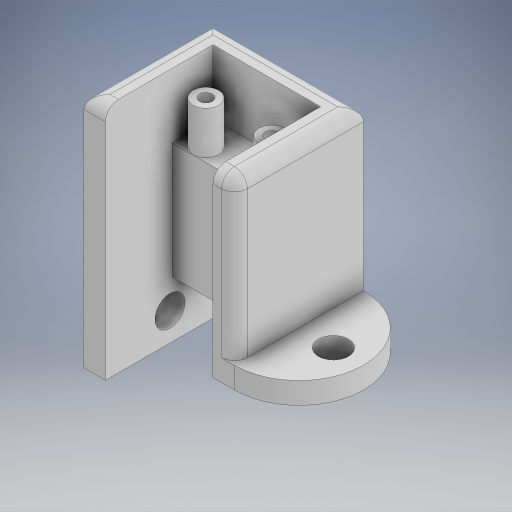
# Autodesk Inventor part: imu_mount
Saved by Autodesk Inventor 2024 (Build 280153000, 153)
## iProperties
Created: 2025-01-15
Part Number: imu_mount
Material: Generic
Document SubType Name: Modeling
Designer: Alex
Density: 1 g/cm^3
Appearance: Default
Author: Alex
Autodesk Inventor part; units mm, degrees
ref_plane "YZ Plane" through (0, 0, 0) normal (1, 0, 0) x (0, 1, 0)
ref_plane "XZ Plane" through (0, 0, 0) normal (0, 1, 0) x (-1, 0, 0)
ref_plane "XY Plane" through (0, 0, 0) normal (0, 0, 1) x (1, 0, 0)
sketch "Sketch1" plane through (0, 0, 0) normal (0, 1, 0) x (-1, 0, 0)
  line L0 (0, 0) -> (35, 0) construction
  line L1 (35, 0) -> (35, -30)
  line L2 (35, -30) -> (0, -30)
  line L3 (0, -30) -> (0, 0)
  line L4 (30, -25) -> (30, -5)
  line L5 (30, -5) -> (5, -5) construction
  line L6 (5, -5) -> (5, -25)
  line L7 (5, -25) -> (30, -25)
  line L8 (30, -5) -> (30, 0)
  line L9 (5, -5) -> (5, 0)
  line L10 (5, 0) -> (0, 0)
  line L11 (30, 0) -> (35, 0)
  dimension "d0" = 35
  dimension "d1" = 30
  dimension "d2" = 5
  constraints: 24 end point, 4 parallel, 4 perpendicular, 2 collinear, 2 point on line, 1 horizontal, 3 other
  measures "d0" distance between parallel lines of L3 L1
  measures "d1" distance between parallel lines of L2 L0
  measures "d2" distance between parallel lines of L1 L4
extrude "Extrusion1" add sketch "Sketch1" along normal blind 42
sketch "Sketch2" plane through (0, 0, 0) normal (0, 1, 0) x (-1, 0, 0)
  line L0 (30, 0) -> (30, -25) projected
  line L1 (5, -25) -> (5, 0) projected
  line L2 (30, -25) -> (5, -25)
  line L3 (5, -25) -> (5, -15.519)
  line L4 (5, -15.519) -> (30, -15.519)
  line L5 (30, -15.519) -> (30, -25)
  point P0 (0, 0)
  dimension "d5" = 9.481
  constraints: 8 end point, 2 parallel, 1 horizontal, 1 perpendicular, 1 point on line
  measures "d5" distance between parallel lines of L2 L4
extrude "Extrusion2" add sketch "Sketch2" along normal blind 27
sketch "Sketch3" plane through (0, 27, 0) normal (0, 1, 0) x (1, 0, 0)
  circle A0 centre (-25.15, 18.519) radius 1.5
  line L0 (-30, 0) -> (-30, 15.519) projected
  circle A1 centre (-25.15, 18.519) radius 3
  line L1 (-30, 15.519) -> (-5, 15.519) projected
  line L2 (-17.5, 15.519) -> (-17.5, 30) construction
  line L3 (0, 30) -> (-35, 30) construction
  circle A2 centre (-9.85, 18.519) radius 1.5
  circle A3 centre (-9.85, 18.519) radius 3
  point P0 (0, 0)
  dimension "d8" = 3
  dimension "d9" = 4.85
  dimension "d10" = 6
  constraints: 4 centre point, 2 coincident, 2 end point, 2 midpoint, 2 symmetric about line, 1 tangent, 2 other
  measures "d8" diameter of A0
  measures "d9" distance from line of L0 A0.centre
  measures "d10" diameter of A1
extrude "Extrusion3" add sketch "Sketch3" along normal blind 10
sketch "Sketch4" plane through (0, 0, 0) normal (0, -1, 0) x (1, 0, 0)
  line L0 (-35, -30) -> (-35, 0) projected
  line L1 (0, -30) -> (-35, -30) projected
  line L2 (-35, 0) -> (-30, 0)
  line L3 (-30, 0) -> (-30, -30)
  line L4 (-30, -30) -> (-35, -30)
  line L5 (-35, -30) -> (-35, 0)
  line L6 (-30, 0) -> (-30, -15.519) projected
  point P0 (0, 0)
  constraints: 8 end point, 2 parallel, 2 point on line, 1 horizontal, 1 perpendicular
extrude "Extrusion4" add sketch "Sketch4" along normal blind 13.047
sketch "Sketch5" plane through (0, 0, 0) normal (1, 0, 0) x (0, 0, -1)
  line L0 (15.519, 0) -> (0, 0) projected
  line L1 (30, 0) -> (30, 42) projected
  line L2 (0, 0) -> (30, 0)
  line L3 (30, 0) -> (30, 5)
  line L4 (30, 5) -> (0, 5)
  line L5 (0, 5) -> (0, 0)
  dimension "d15" = 5
  constraints: 8 end point, 2 parallel, 1 horizontal, 1 perpendicular, 1 point on line
  measures "d15" distance between parallel lines of L2 L4
extrude "Extrusion5" add sketch "Sketch5" along normal blind 15
sketch "Sketch6" plane through (0, 5, 0) normal (0, 1, 0) x (1, 0, 0)
  circle A0 centre (8, 7) radius 3.5 construction
  circle A1 centre (8, 23) radius 3.5 construction
  line L0 (8, 7) -> (8, 23) construction
  line L1 (8, 15) -> (15, 15) construction
  line L2 (15, 0) -> (15, 30) construction
  line L3 (15, 30) -> (15, 0) construction
  line L4 (0, 30) -> (15, 30) construction
  circle A2 centre (8, 15) radius 3.5
  point P0 (0, 0)
  dimension "d18" = 7
  dimension "d19" = 7
  dimension "d20" = 7
  dimension "d21" = 7
  dimension "d25" = 7
  constraints: 4 end point, 3 centre point, 2 midpoint, 2 perpendicular, 1 coincident
  measures "d18" diameter of A0
  measures "d19" diameter of A1
  measures "d20" distance from line of L2 L0.end
  measures "d21" distance from line of L4 L0.end
  measures "d25" diameter of A2
extrude "Extrusion6" cut sketch "Sketch6" against normal up to surface (5 mm away) from surface at 0
sketch "Sketch7" plane through (-35, 42, -30) normal (-1, 0, 0) x (0, 0, 1)
  point P0 (30, -42)
sketch "Sketch8" plane through (-35, 42, -30) normal (-1, 0, 0) x (0, 0, 1)
  line L0 (0, -55.047) -> (0, 0) projected
  line L1 (30, -55.047) -> (30, 0) projected
  line L2 (0, -55.047) -> (30, -55.047) construction
  line L3 (30, -55.047) -> (30, -42.047) construction
  line L4 (30, -42.047) -> (0, -42.047) construction
  line L5 (0, -42.047) -> (0, -55.047) construction
  circle A0 centre (15, -48.547) radius 3.5
  point P0 (30, -42)
  dimension "d24" = 13
  dimension "d26" = 7
  dimension "d27" = 6.5
  dimension "d28" = 15
  constraints: 8 end point, 2 parallel, 1 centre point, 1 horizontal, 1 perpendicular, 1 point on line
  measures "d24" distance of L3.end L2.end
  measures "d26" diameter of A0
  measures "d27" distance from line of L2 A0.centre
  measures "d28" distance from line of L0 A0.centre
extrude "Extrusion7" cut sketch "Sketch8" against normal up to next
fillet "Fillet1" radius 3 6 edges at (0, 42, -15) (0, 23.5, 0) (-35, 42, -15) (-17.5, 42, -30) (-2.5, 42, 0) (-32.5, 42, 0)
fillet "Fillet2" radius 15 2 edges at (15, 2.5, 0) (15, 2.5, -30)
equation "\"d21\" = d20"
body "Solid1"
